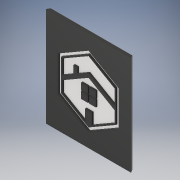
# Autodesk Inventor part: BA03
Saved by Autodesk Inventor 2017 (Build 210142000, 142)
## iProperties
Created: 2018-10-18
Part Number: BA03
Material: ABS Plastic
Document SubType Name: Modeling
Designer: Dell
Density: 1.06 g/cm^3
Appearance: Smooth - Black
Author: Dell
Autodesk Inventor part; units mm, degrees
ref_plane "YZ Plane" through (0, 0, 0) normal (1, 0, 0) x (0, 1, 0)
ref_plane "XZ Plane" through (0, 0, 0) normal (0, 1, 0) x (-1, 0, 0)
ref_plane "XY Plane" through (0, 0, 0) normal (0, 0, 1) x (1, 0, 0)
sketch "Sketch1" plane through (0, 0, 0) normal (0, 0, 1) x (1, 0, 0)
  line L0 (0, 0) -> (292.1, 0)
  line L1 (292.1, 0) -> (292.1, -355.6)
  line L2 (292.1, -355.6) -> (0, -355.6)
  line L3 (0, -355.6) -> (0, 0)
  dimension "d0" = 292.1
  dimension "d1" = 355.6
  constraints: 8 end point, 2 parallel, 1 horizontal, 1 perpendicular
  measures "d0" distance of L1.end L2.end
  measures "d1" distance of L0.end L1.end
extrude "Extrusion1" add sketch "Sketch1" along normal blind 10
sketch "Sketch2" plane through (0, 0, 0) normal (0, 1, 0) x (1, 0, 0)
  line L0 (292.1, -10) -> (0, -10) projected
  line L1 (0, -10) -> (-5.7735, -10)
  line L2 (-5.7735, -10) -> (0, 0)
  line L3 (0, 0) -> (0, -10) projected
  line L4 (0, 0) -> (0, -10) projected
  line L5 (0, -10) -> (0, 0)
  line L6 (292.1, -10) -> (297.8735, -10)
  line L7 (292.1, 0) -> (292.1, -10) projected
  line L8 (297.8735, -10) -> (292.1, 0)
  line L9 (292.1, 0) -> (292.1, -10)
  dimension "d4" = 30
  dimension "d5" = 60
  constraints: 12 end point, 2 collinear, 2 horizontal
  measures "d4" angle of L3 L2
  measures "d5" angle of L6 L8
extrude "Extrusion2" add sketch "Sketch2" against normal blind 355.6
sketch "Sketch4" plane through (0, 0, 10) normal (0, 0, 1) x (1, 0, 0)
  line L0 (21.05, -52.8) -> (271.05, -52.8) construction
  line L1 (271.05, -52.8) -> (271.05, -302.8) construction
  line L2 (271.05, -302.8) -> (21.05, -302.8) construction
  line L3 (21.05, -302.8) -> (21.05, -52.8) construction
  line L4 (146.05, -52.8) -> (254.3032, -115.3)
  line L5 (254.3032, -115.3) -> (254.3032, -240.3)
  line L6 (254.3032, -240.3) -> (146.05, -302.8)
  line L7 (146.05, -302.8) -> (37.7968, -240.3)
  line L8 (37.7968, -240.3) -> (37.7968, -115.3)
  line L9 (37.7968, -115.3) -> (146.05, -52.8)
  line L10 (146.05, -64.5779) -> (244.1032, -121.189)
  line L11 (244.1032, -121.189) -> (244.1032, -234.411)
  line L12 (244.1032, -234.411) -> (146.05, -291.0221)
  line L13 (146.05, -291.0221) -> (47.9968, -234.411)
  line L14 (47.9968, -234.411) -> (47.9968, -121.189)
  line L15 (47.9968, -121.189) -> (146.05, -64.5779)
  line L16 (146.05, -69.4854) -> (239.8532, -123.6427) construction
  line L17 (239.8532, -123.6427) -> (239.8532, -231.9573) construction
  line L18 (239.8532, -231.9573) -> (146.05, -286.1146) construction
  line L19 (146.05, -286.1146) -> (52.2468, -231.9573) construction
  line L20 (52.2468, -231.9573) -> (52.2468, -123.6427) construction
  line L21 (52.2468, -123.6427) -> (146.05, -69.4854) construction
  line L22 (52.2468, -176.1427) -> (92.2468, -153.0487)
  line L23 (92.2468, -153.0487) -> (92.2468, -124.5487)
  line L24 (92.2468, -124.5487) -> (106.2468, -124.5487)
  line L25 (106.2468, -124.5487) -> (106.2468, -144.9658)
  line L26 (106.2468, -144.9658) -> (146.05, -121.9854)
  line L27 (146.05, -121.9854) -> (239.8532, -176.1427)
  line L28 (239.8532, -176.1427) -> (239.8532, -123.6427)
  line L29 (239.8532, -123.6427) -> (146.05, -69.4854)
  line L30 (146.05, -69.4854) -> (52.2468, -123.6427)
  line L31 (52.2468, -176.1427) -> (52.2468, -123.6427)
  line L32 (52.2468, -231.9573) -> (134.05, -279.1864)
  line L33 (134.05, -279.1864) -> (134.05, -239.1146)
  line L34 (134.05, -239.1146) -> (158.05, -239.1146)
  line L35 (158.05, -239.1146) -> (158.05, -279.1864)
  line L36 (158.05, -279.1864) -> (239.8532, -231.9573)
  line L37 (239.8532, -231.9573) -> (239.8532, -191.1427)
  line L38 (239.8532, -191.1427) -> (146.05, -136.9854)
  line L39 (146.05, -136.9854) -> (52.2468, -191.1427)
  line L40 (52.2468, -191.1427) -> (52.2468, -231.9573)
  line L41 (119.8, -165.1146) -> (172.3, -165.1146) construction
  line L42 (172.3, -165.1146) -> (172.3, -216.1146) construction
  line L43 (172.3, -216.1146) -> (119.8, -216.1146) construction
  line L44 (119.8, -216.1146) -> (119.8, -165.1146) construction
  line L45 (119.8, -216.1146) -> (143.8, -216.1146)
  line L46 (143.8, -216.1146) -> (143.8, -192.1146)
  line L47 (143.8, -192.1146) -> (119.8, -192.1146)
  line L48 (119.8, -192.1146) -> (119.8, -216.1146)
  line L49 (119.8, -165.1146) -> (143.8, -165.1146)
  line L50 (143.8, -165.1146) -> (143.8, -189.1146)
  line L51 (143.8, -189.1146) -> (119.8, -189.1146)
  line L52 (119.8, -189.1146) -> (119.8, -165.1146)
  line L53 (172.3, -165.1146) -> (148.3, -165.1146)
  line L54 (148.3, -165.1146) -> (148.3, -189.1146)
  line L55 (148.3, -189.1146) -> (172.3, -189.1146)
  line L56 (172.3, -189.1146) -> (172.3, -165.1146)
  line L57 (172.3, -216.1146) -> (148.3, -216.1146)
  line L58 (148.3, -216.1146) -> (148.3, -192.1146)
  line L59 (148.3, -192.1146) -> (172.3, -192.1146)
  line L60 (172.3, -192.1146) -> (172.3, -216.1146)
  line L61 (-5.7735, 0) -> (297.8735, 0) projected
  line L62 (-5.7735, 0) -> (-5.7735, -355.6) projected
  point P0 (0, 0)
  point P1 (146.05, -177.8)
  point P2 (146.05, -239.1146)
  point P3 (146.05, -165.1146)
  point P4 (271.05, -177.8)
  point P5 (21.05, -177.8)
  point P6 (-5.7735, -177.8)
  point P7 (146.05, 0)
  dimension "d19" = 250
  dimension "d20" = 10.2
  dimension "d21" = 4.25
  dimension "d22" = 52.5
  dimension "d23" = 40
  dimension "d24" = 14
  dimension "d25" = 28.5
  dimension "d26" = 15
  dimension "d27" = 24
  dimension "d28" = 47
  dimension "d29" = 23
  dimension "d30" = 51
  dimension "d31" = 52.5
  dimension "d32" = 24
  dimension "d33" = 24
  dimension "d34" = 24
  dimension "d35" = 24
  dimension "d36" = 24
  dimension "d37" = 24
  dimension "d38" = 24
  dimension "d39" = 24
  constraints: 114 end point, 15 parallel, 9 perpendicular, 8 midpoint, 8 point on line, 6 vertical alignment, 5 horizontal, 4 collinear, 2 vertical, 1 horizontal alignment, 24 other
  measures "d19" distance of L0.start L1.start
  measures "d20" distance between parallel lines of L9 L15
  measures "d21" distance between parallel lines of L15 L21
  measures "d22" distance of L22.start L20.end
  measures "d23" distance between parallel lines of L20 L23
  measures "d24" distance of L24.start L24.end
  measures "d25" distance of L23.start L24.start
  measures "d26" distance of L26.end L39.start
  measures "d27" distance between parallel lines of L35 L33
  measures "d28" distance from line of L18.end L34
  measures "d29" distance between parallel lines of L34 L43
  measures "d30" distance of L45.start L52.end
  measures "d31" distance of L52.end L56.end
  measures "d32" distance of L47.end L47.start
  measures "d33" distance of L47.start L45.end
  measures "d34" distance of L50.end L52.start
  measures "d35" distance of L49.end L50.end
  measures "d36" distance of L55.end L55.start
  measures "d37" distance of L55.start L53.end
  measures "d38" distance of L58.end L60.start
  measures "d39" distance of L58.start L58.end
extrude "Extrusion4" cut sketch "Sketch4" against normal blind 5
body "Solid1"
